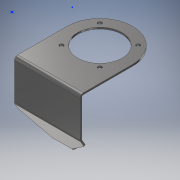
# Autodesk Inventor part: Lamiera supporto motore
Saved by Autodesk Inventor 2018 (Build 220112000, 112)
## iProperties
Created: 2020-06-04
Part Number: Lamiera supporto motore
Material: Acciaio inossidabile
Document SubType Name: Lamiera
Designer: Francesco
Density: 8 g/cm^3
Sheet Metal Rule: Default_mm
Appearance: Semilucidato
Mass: 2829.96 g
Surface Area: 1504.71 cm^2
Volume: 353.745 cm^3
Author: Francesco
Autodesk Inventor part; units mm, degrees
ref_plane "YZ Plane" through (0, 0, 0) normal (1, 0, 0) x (0, 1, 0)
ref_plane "XZ Plane" through (0, 0, 0) normal (0, 1, 0) x (-1, 0, 0)
ref_plane "XY Plane" through (0, 0, 0) normal (0, 0, 1) x (1, 0, 0)
sketch "Schizzo1" plane through (0, 0, 0) normal (0, 0, 1) x (1, 0, 0)
  line L0 (100, 75) -> (100, -75)
  line L1 (100, -75) -> (-100, -75)
  line L2 (-100, -75) -> (-100, 75)
  line L3 (-100, 75) -> (100, -75) construction
  line L4 (100, 75) -> (-100, -75) construction
  arc A0 (100, 75) -> (-100, 75) centre (0, 75) ccw
  circle A1 centre (0, 75) radius 67.5
  point P0 (0, 0)
  point P1 (0, 0)
  dimension "d0" = 200
  dimension "d1" = 150
  dimension "d3" = 100
  dimension "d4" = 135
  measures "d0" distance of L0.end L1.end
  measures "d1" distance of L0.start L0.end
  measures "d3" radius of A0
  measures "d4" diameter of A1
extrude "Piano2" add sketch "Schizzo1" along normal blind 5
sketch "Schizzo2" plane through (-100, -80, -5) normal (0, -1, 0) x (1, 0, 0)
  line L0 (200, 0) -> (0, 0)
  line L1 (0, 0) -> (0, -110)
  line L2 (0, -110) -> (200, -110)
  line L3 (200, -110) -> (200, 0)
  constraints: 6 end point, 1 horizontal, 1 perpendicular, 1 vertical
edge flange "Flangia1" height 120 angle 90 thickness 5 bend radius 5 thickness toward (0, -1, 0) relief tear relief width 5 relief depth 2.5 edges at (0, -75, 0) wall of the first edge with corners at (100, -80, -5) (-100, -80, -5) (-100, -80, -115) (100, -80, -115)
bend "Piega (Bend)1"
corner "Angolo1"
sketch "Schizzo3" plane through (-100, -79.3301, -117.5) normal (0, -0.8660254, -0.5) x (1, 0, 0)
  line L0 (200, 0) -> (0, 0)
  line L1 (0, 0) -> (0, -87.3205)
  line L2 (0, -87.3205) -> (200, -87.3205)
  line L3 (200, -87.3205) -> (200, 0)
  constraints: 6 end point, 1 horizontal, 1 perpendicular, 1 vertical
edge flange "Flangia2" height 90 angle 30 thickness 5 bend radius 5 thickness toward (0, -0.8660254, -0.5) relief tear relief width 5 relief depth 2.5 edges at (0, -80, -115) wall of the first edge with corners at (100, -79.3301, -117.5) (-100, -79.3301, -117.5) (-100, -35.6699, -193.1218) (100, -35.6699, -193.1218)
bend "Piega (Bend)2"
corner "Angolo2"
sketch "Schizzo5" plane through (0, 0, 5) normal (0, 0, 1) x (1, 0, 0)
  circle A0 centre (58.3363, 133.3363) radius 6 projected
  circle A1 centre (-58.3363, 133.3363) radius 6 projected
  circle A2 centre (-58.3363, 16.6637) radius 6 projected
  circle A3 centre (58.3363, 16.6637) radius 6 projected
  point P0 (0, 0)
  constraints: 4 coincident
hole "Foro1" at (-58.3363, 133.3363, 5) at (58.3363, 133.3363, 5) at (58.3363, 16.6637, 5) at (-58.3363, 16.6637, 5) direction (0, 0, -1) diameter 12 end through all
sketch "Schizzo6" plane through (-100, -35.6699, -193.1218) normal (0, 0.8660254, 0.5) x (1, 0, 0)
  line L0 (200, 0) -> (0, 0) projected
  line L1 (100, 0) -> (130, 0)
  line L2 (130, 0) -> (200, -67.3205)
  line L3 (100, 0) -> (70, 0)
  line L4 (0, 0) -> (0, -87.3205) projected
  line L5 (0, -67.3205) -> (70, 0)
  line L6 (200, -67.3205) -> (200, 19.9941)
  line L7 (200, 19.9941) -> (0, 19.9941)
  line L8 (0, 19.9941) -> (0, -67.3205)
  point P0 (100, -149.4134)
  point P1 (200, -87.3205)
  dimension "d43" = 20
  dimension "d44" = 30
  dimension "d45" = 30
  dimension "d46" = 20
  constraints: 14 end point, 3 point on line, 1 collinear, 1 midpoint, 1 perpendicular
  measures "d43" distance of point (200, -87.321) L2.end
  measures "d44" distance of L1.start L1.end
  measures "d45" distance of L1.start L3.end
  measures "d46" distance of L4.end L5.start
extrude "Taglia1" cut sketch "Schizzo6" against normal blind 5
sketch "Schizzo7" plane through (-30, -31.3397, -195.6218) normal (0, 0, -1) x (-1, 0, 0)
  line L0 (-60, 0) -> (0, 0)
  line L1 (0, 0) -> (0, 24.2265)
  line L2 (0, 24.2265) -> (-60, 24.2265)
  line L3 (-60, 24.2265) -> (-60, 0)
  constraints: 6 end point, 1 horizontal, 1 perpendicular, 1 vertical
edge flange "Flangia4" height 30 angle 60 thickness 5 bend radius 5 thickness toward (0, 0, -1) relief tear relief width 5 relief depth 2.5 edges at (0, -35.6699, -193.1218) wall of the first edge with corners at (30, -31.3397, -195.6218) (-30, -31.3397, -195.6218) (-30, -7.1132, -195.6218) (30, -7.1132, -195.6218)
bend "Piega (Bend)4"
corner "Angolo4"
fillet "Arrotondamento angolo1" radius 5 2 edges at (30, -7.1132, -198.1218) (-30, -7.1132, -198.1218)
sketch "Schizzo8" plane through (-100, -80, -5) normal (0, 1, 0) x (1, 0, 0)
  circle A0 centre (190, 90) radius 2.5 projected
  point P0 (100, -5)
  constraints: 1 coincident
hole "Foro2" at (90, -80, -95) direction (0, -1, 0) diameter 10 end through all
equation "\"d41\" = Spessore"
equation "\"d47\" = Spessore"
equation "\"d65\" = Spessore"
equation "\"d5\" = Spessore"
equation "\"d6\" = LarghezzaScaricoPiega"
equation "\"d7\" = ProfonditàScaricoPiega"
equation "\"d8\" = ResiduoMinimo"
equation "\"d9\" = RaggioTransizione"
equation "\"d12\" = RaggioPiega"
equation "\"d13\" = DimensioniScaricoAngolo"
equation "\"d14\" = DimensioneGioco"
equation "\"d15\" = Dimensione_raggio_Jacobi"
equation "\"d16\" = LarghezzaScaricoPiega"
equation "\"d17\" = ProfonditàScaricoPiega"
equation "\"d18\" = ResiduoMinimo"
equation "\"d19\" = RaggioTransizione"
equation "\"d22\" = RaggioPiega"
equation "\"d23\" = DimensioniScaricoAngolo"
equation "\"d24\" = DimensioneGioco"
equation "\"d25\" = Dimensione_raggio_Jacobi"
equation "\"d49\" = LarghezzaScaricoPiega"
equation "\"d50\" = ProfonditàScaricoPiega"
equation "\"d51\" = ResiduoMinimo"
equation "\"d52\" = RaggioTransizione"
equation "\"d55\" = RaggioPiega"
equation "\"d56\" = DimensioniScaricoAngolo"
equation "\"d57\" = DimensioneGioco"
equation "\"d58\" = Dimensione_raggio_Jacobi"
equation "\"RaggioPiega\" = Spessore"
equation "\"LarghezzaScaricoPiega\" = Spessore"
equation "\"ProfonditàScaricoPiega\" = 0.5 * Spessore"
equation "\"RaggioTransizione\" = RaggioPiega"
equation "\"Dimensione_raggio_Jacobi\" = RaggioPiega"
equation "\"DimensioneGioco\" = Spessore"
equation "\"Spessore\" = 5"
equation "\"ResiduoMinimo\" = 10"
equation "\"DimensioniScaricoAngolo\" = 20"
